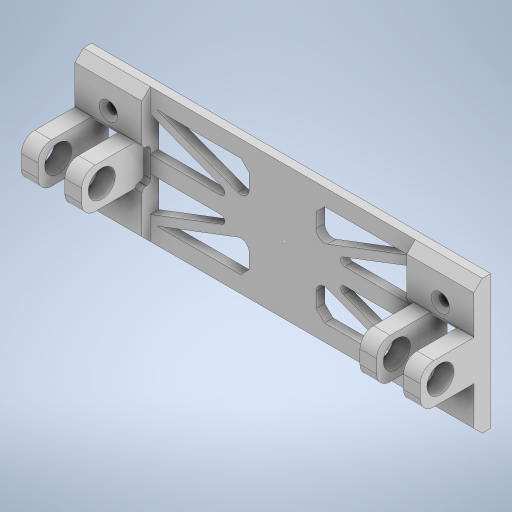
# Autodesk Inventor part: belt tensioner base
Saved by Autodesk Inventor 2023 (Build 270158030, 158C)
## iProperties
Created: 2022-10-08
Part Number: belt tensioner base
Material: Generic
Document SubType Name: Modeling
Designer: rm0990889
Density: 1 g/cm^3
Appearance: Default
Author: rm0990889
Autodesk Inventor part; units mm, degrees
ref_plane "YZ Plane" through (0, 0, 0) normal (1, 0, 0) x (0, 1, 0)
ref_plane "XZ Plane" through (0, 0, 0) normal (0, 1, 0) x (-1, 0, 0)
ref_plane "XY Plane" through (0, 0, 0) normal (0, 0, 1) x (1, 0, 0)
sketch "Sketch1" plane through (0, 0, 0) normal (0, 0, 1) x (1, 0, 0)
  line L0 (0, 10.4492) -> (0, -5.5867)
  line L1 (-50.8, 47.0224) -> (-50.8, -22.5801)
  line L2 (49.53, -22.5801) -> (49.53, 35.616)
  line L3 (-76.2, 44.5628) -> (-76.2, -34.6645)
  line L4 (74.93, 44.5628) -> (74.93, -34.6645)
  line L5 (-76.2, 25.4) -> (74.93, 25.4)
  line L6 (49.53, 35.616) -> (49.53, 84.3028)
  line L7 (-50.8, -22.5801) -> (-50.8, -93.3226)
  line L8 (49.53, -22.5801) -> (49.53, -89.9068)
  line L9 (-76.2, -25.4) -> (74.93, -25.4)
  circle A0 centre (-63.5, 12.7) radius 1.905
  circle A1 centre (-63.5, -12.7) radius 1.905
  circle A2 centre (62.23, -12.7) radius 1.905
  circle A3 centre (62.23, 12.7) radius 1.905
  point P0 (0, 0)
  point P1 (49.53, -25.4)
  point P2 (49.53, 25.4)
  point P3 (-50.8, -25.4)
  point P4 (-50.8, 25.4)
  dimension "d0" = 100.33
  dimension "d1" = 50.8
  dimension "d2" = 25.4
  dimension "d3" = 25.4
  dimension "d4" = 50.8
  dimension "d5" = 25.4
  dimension "d6" = 3.81
  dimension "d7" = 3.81
  dimension "d8" = 3.81
  dimension "d9" = 3.81
  dimension "d10" = 12.7
  dimension "d11" = 12.7
  dimension "d12" = 12.7
  dimension "d13" = 12.7
  dimension "d14" = 12.7
  dimension "d15" = 12.7
  dimension "d16" = 12.7
  dimension "d17" = 12.7
  constraints: 20 end point, 9 vertical, 4 centre point, 4 point on line, 2 perpendicular
  measures "d0" distance between parallel lines of L2 L1
  measures "d1" distance between parallel lines of L1 L0
  measures "d2" distance between parallel lines of L4 L2
  measures "d3" distance between parallel lines of L1 L3
  measures "d4" distance between parallel lines of L9 L5
  measures "d5" distance from line of L5 point (0, 0)
  measures "d6" diameter of A0
  measures "d7" diameter of A1
  measures "d8" diameter of A2
  measures "d9" diameter of A3
  measures "d10" distance from line of L5 A0.centre
  measures "d11" distance from line of L9 A1.centre
  measures "d12" distance from line of L9 A2.centre
  measures "d13" distance from line of L5 A3.centre
  measures "d14" distance from line of L4 A3.centre
  measures "d15" distance from line of L4 A2.centre
  measures "d16" distance from line of L3 A1.centre
  measures "d17" distance from line of L3 A0.centre
extrude "Extrusion1" add sketch "Sketch1" along normal blind 6.35 contours L1 L7 L9 L3 L5 | L5 L4 L9 L8 L2
chamfer "Chamfer1" distance 3.175 angle 45 4 edges at (-63.5, -25.4, 6.35) (62.23, -25.4, 6.35) (62.23, 25.4, 6.35) (-63.5, 25.4, 6.35)
sketch "Sketch2" plane through (74.93, -25.4, 0) normal (1, 0, 0) x (0, 0, -1)
  line L0 (-3.1477, 31.75) -> (-3.1477, 19.05)
  line L1 (0, 50.8) -> (-3.175, 50.8) projected
  line L2 (-3.1477, 31.75) -> (-6.35, 31.75)
  line L3 (-6.35, 31.75) -> (-6.35, 19.05)
  line L4 (-6.35, 3.175) -> (-6.35, 47.625) projected
  line L5 (-3.1477, 19.05) -> (-6.35, 19.05)
  point P0 (0, 25.4)
  dimension "d23" = 12.7
  dimension "d24" = 19.05
  constraints: 8 end point, 1 horizontal, 1 perpendicular, 1 point on line, 1 vertical
  measures "d23" distance of L0.start L0.end
  measures "d24" distance from line of L1 L0.start
extrude "Extrusion2" cut sketch "Sketch2" against normal blind 203.2
fillet "Fillet1" radius 1.524 8 edges at (-63.5, 6.35, 3.1477) (-63.5, 6.35, 6.35) (62.23, 6.35, 6.35) (62.23, 6.35, 3.1477) (62.23, -6.35, 3.1477) (62.23, -6.35, 6.35) (-63.5, -6.35, 3.1477) (-63.5, -6.35, 6.35)
chamfer "Chamfer2" distance 1.524 angle 45 4 edges at (-65.405, 12.7, 6.35) (60.325, 12.7, 6.35) (60.325, -12.7, 6.35) (-65.405, -12.7, 6.35)
sketch "Sketch3" plane through (0, 0, 0) normal (0, 0, -1) x (-1, 0, 0)
  line L0 (-74.93, 25.4) -> (-49.53, 25.4) projected
  line L1 (50.8, -25.4) -> (50.8, 25.4) projected
  line L2 (-49.53, 25.4) -> (50.8, 25.4)
  line L3 (-49.53, 25.4) -> (-49.53, -25.4) projected
  line L4 (50.8, -25.4) -> (-49.53, -25.4)
  line L5 (-49.53, -4.826) -> (-49.53, 4.826) projected
  line L6 (50.8, 4.826) -> (50.8, -4.826) projected
  line L7 (-49.53, -7.874) -> (-49.53, -22.225) projected
  line L8 (-46.99, 19.05) -> (-16.3725, 7.3597)
  line L9 (-49.53, 22.225) -> (-49.53, 7.874) projected
  line L10 (-49.53, 16.51) -> (-22.3253, 6.1227)
  line L11 (-46.99, -19.05) -> (-16.3725, -7.3597)
  line L12 (-49.53, -16.51) -> (-22.3253, -6.1227)
  line L13 (0.635, 25.4) -> (0.635, -25.4)
  line L14 (48.26, 19.05) -> (17.6425, 7.3597)
  line L15 (50.8, 16.51) -> (23.5953, 6.1227)
  line L16 (50.8, -16.51) -> (23.5953, -6.1227)
  line L17 (48.26, -19.05) -> (17.6425, -7.3597)
  line L18 (-12.065, 15.875) -> (-12.065, 10.3258)
  line L19 (-12.065, -10.3258) -> (-12.065, -15.875)
  line L20 (13.335, 15.875) -> (13.335, 10.3258)
  line L21 (13.335, -10.3258) -> (13.335, -15.875)
  line L22 (-49.53, 3.175) -> (-22.8689, 3.175)
  line L23 (24.1389, 3.175) -> (50.8, 3.175)
  line L24 (-49.53, -3.175) -> (-22.8689, -3.175)
  line L25 (24.1389, -3.175) -> (50.8, -3.175)
  arc A0 (-16.3725, 7.3597) -> (-12.065, 10.3258) centre (-15.24, 10.3258) ccw
  arc A1 (-12.065, -10.3258) -> (-16.3725, -7.3597) centre (-15.24, -10.3258) ccw
  arc A2 (13.335, 10.3258) -> (17.6425, 7.3597) centre (16.51, 10.3258) ccw
  arc A3 (17.6425, -7.3597) -> (13.335, -10.3258) centre (16.51, -10.3258) ccw
  arc A4 (23.5953, 6.1227) -> (24.1389, 3.175) centre (24.1389, 4.699) ccw
  arc A5 (24.1389, -3.175) -> (23.5953, -6.1227) centre (24.1389, -4.699) ccw
  arc A6 (-22.3253, -6.1227) -> (-22.8689, -3.175) centre (-22.8689, -4.699) ccw
  arc A7 (-22.8689, 3.175) -> (-22.3253, 6.1227) centre (-22.8689, 4.699) ccw
  line L26 (-49.53, 19.05) -> (-15.24, 19.05)
  line L27 (16.51, 19.05) -> (50.8, 19.05)
  line L28 (50.8, -19.05) -> (16.51, -19.05)
  line L29 (-15.24, -19.05) -> (-49.53, -19.05)
  line L30 (-15.24, -19.05) -> (-12.065, -15.875)
  line L31 (16.51, -19.05) -> (13.335, -15.875)
  line L32 (13.335, 15.875) -> (16.51, 19.05)
  line L33 (-15.24, 19.05) -> (-12.065, 15.875)
  point P0 (0, 0)
  point P1 (-12.065, 19.05)
  point P2 (-12.065, -19.05)
  point P3 (13.335, 19.05)
  point P4 (13.335, -19.05)
  point P5 (-14.605, 3.175)
  point P6 (15.875, -3.175)
  point P7 (15.875, 3.175)
  point P8 (-12.065, -5.715)
  point P9 (-12.065, 5.715)
  point P10 (13.335, 5.715)
  point P11 (13.335, -5.715)
  point P12 (-14.605, -3.175)
  dimension "d38" = 2.54
  dimension "d41" = 3.175
  dimension "d42" = 1.524
  dimension "d43" = 3.175
  dimension "d44" = 3.175
  dimension "d45" = 3.175
  dimension "d46" = 3.175
  dimension "d47" = 3.175
  dimension "d48" = 3.175
  dimension "d49" = 3.175
  dimension "d50" = 3.175
  constraints: 54 end point, 29 point on line, 16 point on circle, 16 tangent, 8 centre point, 8 symmetric about line, 6 equal radius, 6 perpendicular, 4 horizontal, 2 midpoint, 2 other
  measures "d41" radius of A0
  measures "d42" radius of A4
  measures "d43" distance of L29.start point (-12.065, -19.05)
  measures "d44" distance of L19.end point (-12.065, -19.05)
  measures "d45" distance of L28.end point (13.335, -19.05)
  measures "d46" distance of L21.end point (13.335, -19.05)
  measures "d47" distance of L20.start point (13.335, 19.05)
  measures "d48" distance of L27.start point (13.335, 19.05)
  measures "d49" distance of L26.end point (-12.065, 19.05)
  measures "d50" distance of L18.start point (-12.065, 19.05)
extrude "Extrusion3" add sketch "Sketch3" against normal blind 3.175 contours L4 L13 L2 L1 L15 A4 L23 L25 A5 L16 | L4 L3 L12 A6 L24 L22 A7 L10 L2 L13
sketch "Sketch4" plane through (-76.2, -4.826, 3.1477) normal (0, 0, 1) x (1, 0, 0)
  point P0 (76.2, 4.826)
sketch "Sketch5" plane through (-76.2, -4.826, 3.1477) normal (0, 0, 1) x (1, 0, 0)
  line L0 (0, -1.524) -> (0, -3.048) projected
  line L1 (0, -3.048) -> (25.4, -3.048) projected
  line L2 (25.4, -3.048) -> (25.4, -1.524) projected
  line L3 (25.4, -1.524) -> (0, -1.524) projected
  line L4 (25.4, -1.524) -> (25.4, 0) projected
  line L5 (25.4, 0) -> (0, 0) projected
  line L6 (0, 0) -> (0, -1.524) projected
  line L7 (0, -1.524) -> (25.4, -1.524) projected
  line L8 (25.4, 9.652) -> (25.4, 11.176) projected
  line L9 (25.4, 11.176) -> (0, 11.176) projected
  line L10 (0, 11.176) -> (0, 9.652) projected
  line L11 (0, 9.652) -> (25.4, 9.652) projected
  line L12 (25.4, 12.7) -> (0, 12.7) projected
  line L13 (0, -3.048) -> (25.4, -3.048) projected
  line L14 (6.35, -3.048) -> (6.35, 12.7)
  line L15 (16.51, 12.7) -> (16.51, -3.048)
  line L16 (0, 0) -> (0, 9.652) projected
  line L17 (22.86, 12.7) -> (22.86, -3.048)
  line L18 (151.13, 30.226) -> (0, 30.226) projected
  line L19 (0, -20.574) -> (151.13, -20.574) projected
  line L20 (0, 12.7) -> (25.4, 12.7)
  line L21 (25.4, -3.048) -> (0, -3.048)
  line L22 (0, 30.226) -> (0, -20.574) projected
  line L23 (75.565, 30.226) -> (75.565, -20.574)
  line L24 (151.13, -1.524) -> (151.13, -3.048)
  line L25 (151.13, -3.048) -> (125.73, -3.048)
  line L26 (125.73, -3.048) -> (125.73, -1.524)
  line L27 (125.73, -1.524) -> (151.13, -1.524)
  line L28 (125.73, -1.524) -> (125.73, 0)
  line L29 (125.73, 0) -> (151.13, 0)
  line L30 (151.13, 0) -> (151.13, -1.524)
  line L31 (151.13, -1.524) -> (125.73, -1.524)
  line L32 (125.73, 9.652) -> (125.73, 11.176)
  line L33 (125.73, 11.176) -> (151.13, 11.176)
  line L34 (151.13, 11.176) -> (151.13, 9.652)
  line L35 (151.13, 9.652) -> (125.73, 9.652)
  line L36 (125.73, 12.7) -> (151.13, 12.7)
  line L37 (151.13, -3.048) -> (125.73, -3.048)
  line L38 (144.78, -3.048) -> (144.78, 12.7)
  line L39 (134.62, 12.7) -> (134.62, -3.048)
  line L40 (151.13, 0) -> (151.13, 9.652)
  line L41 (128.27, 12.7) -> (128.27, -3.048)
  line L42 (151.13, 12.7) -> (125.73, 12.7)
  line L43 (125.73, -3.048) -> (151.13, -3.048)
  point P0 (76.2, 4.826)
  point P1 (144.78, 9.652)
  point P2 (144.78, 0)
  point P3 (128.27, 9.652)
  point P4 (128.27, 0)
  point P5 (134.62, 0)
  point P6 (134.62, 9.652)
  point P7 (22.86, 0)
  point P8 (22.86, 9.652)
  point P9 (16.51, 9.652)
  point P10 (16.51, 0)
  point P11 (6.35, 0)
  point P12 (6.35, 9.652)
  dimension "d53" = 6.35
  dimension "d54" = 10.16
  dimension "d55" = 6.35
  constraints: 52 end point, 20 symmetric about line, 12 point on line, 4 perpendicular, 2 midpoint, 1 horizontal, 1 other
  measures "d53" distance between parallel lines of L16 L14
  measures "d54" distance between parallel lines of L15 L14
  measures "d55" distance between parallel lines of L17 L15
extrude "Extrusion4" add sketch "Sketch5" along normal blind 3.175 contours L16 L11 L14 L5 | L15 L11 L17 L5 | L29 L38 L35 L40 | L29 L41 L35 L39
sketch "Sketch6" plane through (-76.2, -4.826, 3.1477) normal (0, -1, 0) x (1, 0, 0)
  line L0 (6.35, 0) -> (0, 0) projected
  line L1 (6.35, 0) -> (6.35, 3.175) projected
  line L2 (0, 3.175) -> (6.35, 3.175) projected
  line L3 (0, 0) -> (0, 3.175) projected
  line L4 (16.51, 3.175) -> (22.86, 3.175) projected
  line L5 (22.86, 0) -> (16.51, 0) projected
  line L6 (22.86, 0) -> (22.86, 3.175) projected
  line L7 (16.51, 3.175) -> (22.86, 3.175) projected
  line L8 (16.51, 0) -> (16.51, 3.175) projected
  line L9 (134.62, 0) -> (128.27, 0) projected
  line L10 (134.62, 0) -> (134.62, 3.175) projected
  line L11 (128.27, 3.175) -> (134.62, 3.175) projected
  line L12 (128.27, 0) -> (128.27, 3.175) projected
  line L13 (151.13, 0) -> (144.78, 0) projected
  line L14 (151.13, 0) -> (151.13, 3.175) projected
  line L15 (144.78, 3.175) -> (151.13, 3.175) projected
  line L16 (144.78, 0) -> (144.78, 3.175) projected
  line L17 (128.27, 0) -> (134.62, 0) projected
  line L18 (128.27, 0) -> (128.27, 3.175) projected
  line L19 (134.62, 3.175) -> (128.27, 3.175) projected
  line L20 (134.62, 0) -> (134.62, 3.175) projected
  point P0 (76.2, -3.1477)
extrude "Extrusion5" add sketch "Sketch6" along normal blind 3.175
sketch "Sketch7" plane through (-76.2, 4.826, 3.1477) normal (0, 1, 0) x (1, 0, 0)
  line L0 (16.51, 0) -> (22.86, 0) projected
  line L1 (16.51, 0) -> (16.51, -3.175) projected
  line L2 (22.86, -3.175) -> (16.51, -3.175) projected
  line L3 (22.86, 0) -> (22.86, -3.175) projected
  line L4 (0, 0) -> (6.35, 0) projected
  line L5 (0, 0) -> (0, -3.175) projected
  line L6 (6.35, -3.175) -> (0, -3.175) projected
  line L7 (6.35, 0) -> (6.35, -3.175) projected
  line L8 (128.27, 0) -> (134.62, 0) projected
  line L9 (128.27, 0) -> (128.27, -3.175) projected
  line L10 (134.62, -3.175) -> (128.27, -3.175) projected
  line L11 (134.62, 0) -> (134.62, -3.175) projected
  line L12 (144.78, 0) -> (151.13, 0) projected
  line L13 (144.78, 0) -> (144.78, -3.175) projected
  line L14 (151.13, -3.175) -> (144.78, -3.175) projected
  line L15 (151.13, 0) -> (151.13, -3.175) projected
  point P0 (76.2, 3.1477)
extrude "Extrusion6" add sketch "Sketch7" along normal blind 3.175
sketch "Sketch8" plane through (58.42, -4.826, 3.1477) normal (0, 0, 1) x (1, 0, 0)
  line L0 (-118.11, 0) -> (-118.11, 9.652) projected
  line L1 (-128.27, 9.652) -> (-118.11, 9.652) projected
  line L2 (-128.27, 9.652) -> (-128.27, 0) projected
  line L3 (-118.11, 0) -> (-128.27, 0) projected
  line L4 (0, 9.652) -> (0, 0) projected
  line L5 (10.16, 0) -> (0, 0) projected
  line L6 (10.16, 0) -> (10.16, 9.652) projected
  line L7 (0, 9.652) -> (10.16, 9.652) projected
  point P0 (-58.42, 4.826)
extrude "Extrusion7" cut sketch "Sketch8" against normal blind 3.175
sketch "Sketch9" plane through (-59.69, -7.587, 6.3227) normal (-1, 0, 0) x (0, 0, 1)
  circle A0 centre (12.7273, 7.8791) radius 11.303
  line L0 (-6.3227, 2.761) -> (-6.3227, 12.413) projected
  circle A1 centre (12.7273, 7.8791) radius 5.08
  point P0 (-6.3227, 7.587)
  point P1 (0.0273, 15.461)
  dimension "d64" = 22.606
  dimension "d65" = 7.5819
  dimension "d66" = 19.05
  dimension "d70" = 10.16
  constraints: 2 centre point, 1 coincident
  measures "d64" diameter of A0
  measures "d65" vertical distance of point (0.027, 15.461) A0.centre
  measures "d66" distance from line of L0 A0.centre
  measures "d70" diameter of A1
sketch "Sketch10" plane through (-76.2, -4.826, 6.3227) normal (0, 0, 1) x (1, 0, 0)
  line L0 (6.35, 12.413) -> (6.35, -2.761) projected
  line L1 (0, 12.413) -> (6.35, 12.413) projected
  line L2 (0, -2.761) -> (0, 12.413) projected
  line L3 (6.35, -2.761) -> (0, -2.761) projected
  line L4 (16.51, -2.761) -> (16.51, 12.413) projected
  line L5 (22.86, -2.761) -> (16.51, -2.761) projected
  line L6 (22.86, 12.413) -> (22.86, -2.761) projected
  line L7 (16.51, 12.413) -> (22.86, 12.413) projected
  line L8 (134.62, 12.413) -> (134.62, -2.761) projected
  line L9 (128.27, 12.413) -> (134.62, 12.413) projected
  line L10 (128.27, -2.761) -> (128.27, 12.413) projected
  line L11 (134.62, -2.761) -> (128.27, -2.761) projected
  line L12 (144.78, -2.761) -> (144.78, 12.413) projected
  line L13 (151.13, -2.761) -> (144.78, -2.761) projected
  line L14 (151.13, 12.413) -> (151.13, -2.761) projected
  line L15 (144.78, 12.413) -> (151.13, 12.413) projected
  point P0 (76.2, 4.826)
extrude "Extrusion8" add sketch "Sketch10" along normal blind 20.32
fillet "Fillet2" radius 5.08 8 edges at (-73.025, 7.587, 26.6427) (-56.515, 7.587, 26.6427) (-56.515, -7.587, 26.6427) (-73.025, -7.587, 26.6427) (55.245, 7.587, 26.6427) (71.755, 7.587, 26.6427) (71.755, -7.587, 26.6427) (55.245, -7.587, 26.6427)
extrude "Extrusion9" cut sketch "Sketch9" along normal mid plane 406.4 contours A1
equation "\"d44\" = d43"
equation "\"d45\" = d43"
equation "\"d46\" = d45"
equation "\"d47\" = d43"
equation "\"d48\" = d47"
equation "\"d49\" = d43"
equation "\"d50\" = d49"
body "Solid1"
